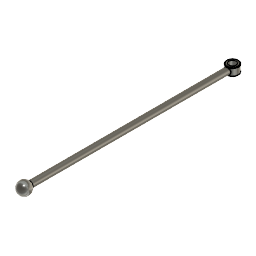
Arm (Autodesk Fusion 360 design; units mm, degrees)
Autodesk Fusion 360 part; units mm, degrees
note: some values were not read from the file. Set by a fixed rule: which sketch regions a step uses.
sketch "Sketch1" plane through (0, 0, 0) normal (0, 0, 1) x (1, 0, 0)
  circle A0 centre (0, 75) radius 1.375
  circle A1 centre (0, 75) radius 2.25
  line L0 (0, 72.75) -> (0, -5)
  circle A2 centre (0, -5) radius 2.5
  line L1 (0, -5) -> (0, -7.5)
  line L2 (1.25, 73.1292) -> (1.25, -2.8349)
  line L3 (-1.25, 73.1292) -> (-1.25, -2.8349)
  dimension "d1" = 2.75
  dimension "d2" = 4.5
  dimension "d3" = 80
  dimension "d4" = 5
  constraint concentric A0 A1
  constraint vertical L0
  constraint coincident L0.end A2.centre
  constraint coincident A2 L1.end
  constraint parallel L0 L1
  constraint coincident A2 L3.end
  constraint coincident A2 L2.end
  constraint coincident A1 L3.start
  constraint coincident A1 L2.start
  constraint coincident A1 L0.start
  measures "d1" diameter of A0
  measures "d2" diameter of A1
  measures "d3" distance of A0.centre L0.end
  measures "d4" diameter of A2
revolve "Revolve1" add sketch "Sketch1" angle 360 about axis through (0, -5, 0) along (0, -1, 0) contours L0 A2 L1 picked at (1.6574, -4.8758)
revolve "Revolve2" add sketch "Sketch1" angle 360 about axis through (0, 72.75, 0) along (0, -1, 0) contours A1 L0 A2 L3
extrude "Extrude1" add sketch "Sketch1" along normal mid plane 3 contours A1
chamfer "Chamfer1" distance 0.2 angle 45 2 edges at (-2.0977, 74.1864, 1.5) (-2.0977, 75.8136, -1.5)
